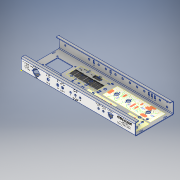
# Autodesk Inventor part: mainChassis
Saved by Autodesk Inventor 2018.3 (Build 223284000, 284)
## iProperties
Created: 2019-02-19
Part Number: mainChassis
Material: Aluminum 6061
Document SubType Name: Sheet Metal
Designer: RCCol
Density: 2.7 g/cm^3
Sheet Metal Rule: .125 thick aluminum
Appearance: Aluminum - Flat
Flat Pattern Width: 34.7497 cm
Flat Pattern Length: 60.325 cm
Flat Pattern Area: 2096.27 cm^2
Sheet Metal Width: 13.681 in
Sheet Metal Length: 23.750 in
Sheet Metal Area: 324.923 in^2
Author: RCCol
Autodesk Inventor part; units mm, degrees
ref_plane "YZ Plane" through (0, 0, 0) normal (1, 0, 0) x (0, 1, 0)
ref_plane "XZ Plane" through (0, 0, 0) normal (0, 1, 0) x (-1, 0, 0)
ref_plane "XY Plane" through (0, 0, 0) normal (0, 0, 1) x (1, 0, 0)
sketch "Sketch1" plane through (0, 0, 0) normal (0, 1, 0) x (-1, 0, 0)
  line L0 (0, 0) -> (-603.25, 0)
  line L1 (-603.25, 0) -> (-603.25, -204.47)
  line L2 (-603.25, -204.47) -> (0, -204.47)
  line L3 (0, -204.47) -> (0, 0)
  line L4 (0, 0) -> (-254, 0)
  line L5 (0, -79.375) -> (0, 0)
  dimension "d0" = 603.25
  dimension "d1" = 204.47
  constraints: 12 end point, 2 horizontal, 2 parallel, 1 perpendicular
  measures "d0" distance of L2.end L1.end
  measures "d1" distance of L1.end L0.end
extrude "Plate1" add sketch "Sketch1" along normal blind 3.175
sketch "Sketch2" plane through (0, 3.175, 0) normal (0, 1, 0) x (1, 0, 0)
  line L0 (41.3, 154.94) -> (117.45, 154.94)
  arc A0 (120.65, 151.74) -> (117.45, 154.94) centre (117.45, 151.74) ccw
  line L1 (41.3, 87.63) -> (117.45, 87.63)
  arc A1 (117.45, 87.63) -> (120.65, 90.83) centre (117.45, 90.83) ccw
  line L2 (38.1, 151.74) -> (38.1, 90.83)
  arc A2 (41.3, 154.94) -> (38.1, 151.74) centre (41.3, 151.74) ccw
  arc A3 (38.1, 90.83) -> (41.3, 87.63) centre (41.3, 90.83) ccw
  circle A4 centre (31.75, 177.5295) radius 1.5
  line L3 (120.65, 151.74) -> (120.65, 90.83)
  circle A5 centre (147.375, 75.2475) radius 1.65
  circle A6 centre (147.375, 164.1475) radius 1.65
  circle A7 centre (185.1575, 138.7475) radius 2.65
  circle A8 centre (185.1575, 178.435) radius 2.65
  circle A9 centre (235.9575, 87.1648) radius 2.65
  circle A10 centre (243.895, 87.1648) radius 2.65
  circle A11 centre (235.9575, 169.7148) radius 2.65
  circle A12 centre (243.895, 169.7148) radius 2.65
  circle A13 centre (259.135, 75.2475) radius 1.65
  circle A14 centre (259.135, 164.1475) radius 1.65
  circle A15 centre (551.549, 97.0569) radius 1.65
  arc A16 (187.6575, 169.4256) -> (182.6575, 169.4256) centre (185.1575, 169.4256) ccw
  arc A17 (182.6575, 164.4256) -> (187.6575, 164.4256) centre (185.1575, 164.4256) ccw
  line L4 (187.6575, 169.4256) -> (187.6575, 164.4256)
  line L5 (182.6575, 169.4256) -> (182.6575, 164.4256)
  arc A18 (187.6575, 90.4475) -> (182.6575, 90.4475) centre (185.1575, 90.4475) ccw
  arc A19 (182.6575, 85.4475) -> (187.6575, 85.4475) centre (185.1575, 85.4475) ccw
  line L6 (187.6575, 90.4475) -> (187.6575, 85.4475)
  line L7 (182.6575, 90.4475) -> (182.6575, 85.4475)
  arc A20 (308.1355, 175.935) -> (308.1355, 180.935) centre (308.1355, 178.435) ccw
  arc A21 (301.1355, 180.935) -> (301.1355, 175.935) centre (301.1355, 178.435) ccw
  line L8 (308.1355, 175.935) -> (301.1355, 175.935)
  line L9 (308.1355, 180.935) -> (301.1355, 180.935)
  arc A22 (243.048, 175.935) -> (243.048, 180.935) centre (243.048, 178.435) ccw
  arc A23 (236.048, 180.935) -> (236.048, 175.935) centre (236.048, 178.435) ccw
  line L10 (243.048, 175.935) -> (236.048, 175.935)
  line L11 (243.048, 180.935) -> (236.048, 180.935)
  arc A24 (298.195, 167.2148) -> (298.195, 172.2148) centre (298.195, 169.7148) ccw
  arc A25 (291.195, 172.2148) -> (291.195, 167.2148) centre (291.195, 169.7148) ccw
  line L12 (298.195, 167.2148) -> (291.195, 167.2148)
  line L13 (298.195, 172.2148) -> (291.195, 172.2148)
  arc A26 (308.1355, 110.435) -> (308.1355, 115.435) centre (308.1355, 112.935) ccw
  arc A27 (301.1355, 115.435) -> (301.1355, 110.435) centre (301.1355, 112.935) ccw
  line L14 (308.1355, 110.435) -> (301.1355, 110.435)
  line L15 (308.1355, 115.435) -> (301.1355, 115.435)
  arc A28 (308.1355, 99.735) -> (308.1355, 104.735) centre (308.1355, 102.235) ccw
  arc A29 (301.1355, 104.735) -> (301.1355, 99.735) centre (301.1355, 102.235) ccw
  line L16 (308.1355, 99.735) -> (301.1355, 99.735)
  line L17 (308.1355, 104.735) -> (301.1355, 104.735)
  arc A30 (243.048, 110.435) -> (243.048, 115.435) centre (243.048, 112.935) ccw
  arc A31 (236.048, 115.435) -> (236.048, 110.435) centre (236.048, 112.935) ccw
  line L18 (243.048, 110.435) -> (236.048, 110.435)
  line L19 (243.048, 115.435) -> (236.048, 115.435)
  arc A32 (243.048, 99.735) -> (243.048, 104.735) centre (243.048, 102.235) ccw
  arc A33 (236.048, 104.735) -> (236.048, 99.735) centre (236.048, 102.235) ccw
  line L20 (243.048, 99.735) -> (236.048, 99.735)
  line L21 (243.048, 104.735) -> (236.048, 104.735)
  arc A34 (298.195, 84.6648) -> (298.195, 89.6648) centre (298.195, 87.1648) ccw
  arc A35 (291.195, 89.6648) -> (291.195, 84.6648) centre (291.195, 87.1648) ccw
  line L22 (298.195, 84.6648) -> (291.195, 84.6648)
  line L23 (298.195, 89.6648) -> (291.195, 89.6648)
  circle A36 centre (237.6, 35.56) radius 15.1
  arc A37 (239.251, 57.4158) -> (238.6557, 58.0111) centre (238.6557, 57.4158) ccw
  arc A38 (238.6557, 53.1089) -> (239.251, 53.7042) centre (238.6557, 53.7042) ccw
  line L24 (239.251, 53.7042) -> (239.251, 57.4158)
  arc A39 (236.5443, 58.0111) -> (235.949, 57.4158) centre (236.5443, 57.4158) ccw
  line L25 (235.949, 53.7042) -> (235.949, 57.4158)
  line L26 (238.6557, 58.0111) -> (236.5443, 58.0111)
  line L27 (238.6557, 53.1089) -> (236.5443, 53.1089)
  arc A40 (235.949, 53.7042) -> (236.5443, 53.1089) centre (236.5443, 53.7042) ccw
  arc A41 (239.251, 17.4158) -> (238.6557, 18.0111) centre (238.6557, 17.4158) ccw
  arc A42 (238.6557, 13.1089) -> (239.251, 13.7042) centre (238.6557, 13.7042) ccw
  line L28 (239.251, 13.7042) -> (239.251, 17.4158)
  arc A43 (236.5443, 18.0111) -> (235.949, 17.4158) centre (236.5443, 17.4158) ccw
  line L29 (235.949, 13.7042) -> (235.949, 17.4158)
  line L30 (238.6557, 18.0111) -> (236.5443, 18.0111)
  line L31 (238.6557, 13.1089) -> (236.5443, 13.1089)
  arc A44 (235.949, 13.7042) -> (236.5443, 13.1089) centre (236.5443, 13.7042) ccw
  circle A45 centre (174.1, 35.56) radius 15.1
  arc A46 (175.751, 57.4158) -> (175.1557, 58.0111) centre (175.1557, 57.4158) ccw
  arc A47 (175.1557, 53.1089) -> (175.751, 53.7042) centre (175.1557, 53.7042) ccw
  line L32 (175.751, 53.7042) -> (175.751, 57.4158)
  arc A48 (173.0443, 58.0111) -> (172.449, 57.4158) centre (173.0443, 57.4158) ccw
  line L33 (172.449, 53.7042) -> (172.449, 57.4158)
  line L34 (175.1557, 58.0111) -> (173.0443, 58.0111)
  line L35 (175.1557, 53.1089) -> (173.0443, 53.1089)
  arc A49 (172.449, 53.7042) -> (173.0443, 53.1089) centre (173.0443, 53.7042) ccw
  arc A50 (175.751, 17.4158) -> (175.1557, 18.0111) centre (175.1557, 17.4158) ccw
  arc A51 (175.1557, 13.1089) -> (175.751, 13.7042) centre (175.1557, 13.7042) ccw
  line L36 (175.751, 13.7042) -> (175.751, 17.4158)
  arc A52 (173.0443, 18.0111) -> (172.449, 17.4158) centre (173.0443, 17.4158) ccw
  line L37 (172.449, 13.7042) -> (172.449, 17.4158)
  line L38 (175.1557, 18.0111) -> (173.0443, 18.0111)
  line L39 (175.1557, 13.1089) -> (173.0443, 13.1089)
  arc A53 (172.449, 13.7042) -> (173.0443, 13.1089) centre (173.0443, 13.7042) ccw
  circle A54 centre (110.6, 35.56) radius 15.1
  arc A55 (112.251, 57.4158) -> (111.6557, 58.0111) centre (111.6557, 57.4158) ccw
  arc A56 (111.6557, 53.1089) -> (112.251, 53.7042) centre (111.6557, 53.7042) ccw
  line L40 (112.251, 53.7042) -> (112.251, 57.4158)
  arc A57 (109.5443, 58.0111) -> (108.949, 57.4158) centre (109.5443, 57.4158) ccw
  line L41 (108.949, 53.7042) -> (108.949, 57.4158)
  line L42 (111.6557, 58.0111) -> (109.5443, 58.0111)
  line L43 (111.6557, 53.1089) -> (109.5443, 53.1089)
  arc A58 (108.949, 53.7042) -> (109.5443, 53.1089) centre (109.5443, 53.7042) ccw
  arc A59 (112.251, 17.4158) -> (111.6557, 18.0111) centre (111.6557, 17.4158) ccw
  arc A60 (111.6557, 13.1089) -> (112.251, 13.7042) centre (111.6557, 13.7042) ccw
  line L44 (112.251, 13.7042) -> (112.251, 17.4158)
  arc A61 (109.5443, 18.0111) -> (108.949, 17.4158) centre (109.5443, 17.4158) ccw
  line L45 (108.949, 13.7042) -> (108.949, 17.4158)
  line L46 (111.6557, 18.0111) -> (109.5443, 18.0111)
  line L47 (111.6557, 13.1089) -> (109.5443, 13.1089)
  arc A62 (108.949, 13.7042) -> (109.5443, 13.1089) centre (109.5443, 13.7042) ccw
  circle A63 centre (47.1, 35.56) radius 15.1
  arc A64 (48.751, 57.4158) -> (48.1557, 58.0111) centre (48.1557, 57.4158) ccw
  arc A65 (48.1557, 53.1089) -> (48.751, 53.7042) centre (48.1557, 53.7042) ccw
  line L48 (48.751, 53.7042) -> (48.751, 57.4158)
  arc A66 (46.0443, 58.0111) -> (45.449, 57.4158) centre (46.0443, 57.4158) ccw
  line L49 (45.449, 53.7042) -> (45.449, 57.4158)
  line L50 (48.1557, 58.0111) -> (46.0443, 58.0111)
  line L51 (48.1557, 53.1089) -> (46.0443, 53.1089)
  arc A67 (45.449, 53.7042) -> (46.0443, 53.1089) centre (46.0443, 53.7042) ccw
  arc A68 (48.751, 17.4158) -> (48.1557, 18.0111) centre (48.1557, 17.4158) ccw
  arc A69 (48.1557, 13.1089) -> (48.751, 13.7042) centre (48.1557, 13.7042) ccw
  line L52 (48.751, 13.7042) -> (48.751, 17.4158)
  arc A70 (46.0443, 18.0111) -> (45.449, 17.4158) centre (46.0443, 17.4158) ccw
  line L53 (45.449, 13.7042) -> (45.449, 17.4158)
  line L54 (48.1557, 18.0111) -> (46.0443, 18.0111)
  line L55 (48.1557, 13.1089) -> (46.0443, 13.1089)
  arc A71 (45.449, 13.7042) -> (46.0443, 13.1089) centre (46.0443, 13.7042) ccw
  circle A72 centre (159.7575, 106.3403) radius 4.8
  circle A73 centre (212.2, 93.5148) radius 4.8
  circle A74 centre (309.5568, 135.335) radius 6.35
  circle A75 centre (234.6268, 135.335) radius 6.35
  circle A76 centre (269.35, 26.9408) radius 1.651
  circle A77 centre (515.9375, 36.5125) radius 9.525
  circle A78 centre (515.3168, 50.7865) radius 1.651
  circle A79 centre (516.5582, 22.2385) radius 1.651
  circle A80 centre (530.225, 142.875) radius 9.525
  circle A81 centre (530.225, 157.1625) radius 1.651
  circle A82 centre (530.225, 128.5875) radius 1.651
  circle A83 centre (425.45, 142.875) radius 9.525
  circle A84 centre (425.45, 157.1625) radius 1.651
  circle A85 centre (425.45, 128.5875) radius 1.651
  circle A86 centre (363.5375, 142.875) radius 9.525
  circle A87 centre (363.5375, 157.1625) radius 1.651
  circle A88 centre (363.5375, 128.5875) radius 1.651
  circle A89 centre (336.55, 37.1475) radius 9.525
  circle A90 centre (336.757, 22.8615) radius 1.651
  circle A91 centre (336.343, 51.4335) radius 1.651
  circle A92 centre (205.85, 26.9408) radius 1.651
  circle A93 centre (78.85, 26.9408) radius 1.651
  circle A94 centre (78.85, 63.0879) radius 1.651
  circle A95 centre (19.05, 63.0879) radius 1.651
  circle A96 centre (142.35, 26.035) radius 1.651
  circle A97 centre (22.225, 20.5908) radius 1.651
  arc A98 (187.6575, 104.4569) -> (182.6575, 104.4569) centre (185.1575, 104.4569) ccw
  arc A99 (182.6575, 99.4569) -> (187.6575, 99.4569) centre (185.1575, 99.4569) ccw
  line L56 (187.6575, 104.4569) -> (187.6575, 99.4569)
  line L57 (182.6575, 104.4569) -> (182.6575, 99.4569)
  circle A100 centre (193.85, 60.5908) radius 1.65
  circle A101 centre (217.85, 60.5908) radius 1.65
  circle A102 centre (205.85, 60.5908) radius 4.826
  circle A103 centre (137.16, 62.3578) radius 1.651
  circle A104 centre (558.8, 109.5375) radius 4.826
  circle A105 centre (558.8, 84.1375) radius 4.826
  circle A106 centre (518.6157, 61.2782) radius 2.3813
  circle A107 centre (529.5939, 97.3765) radius 6.35
  circle A108 centre (563.0654, 61.4489) radius 2.3813
  circle A109 centre (31.75, 159.385) radius 3.175
  circle A110 centre (127, 159.385) radius 3.175
  circle A111 centre (31.75, 83.185) radius 3.175
  circle A112 centre (127, 83.185) radius 3.175
  circle A113 centre (565.8874, 37.1475) radius 9.525
  circle A114 centre (565.8026, 51.4347) radius 1.651
  circle A115 centre (565.9721, 22.8603) radius 1.651
  circle A116 centre (78.85, 35.56) radius 3.2385
  circle A117 centre (142.35, 35.56) radius 3.2385
  circle A118 centre (205.85, 35.56) radius 3.2385
  circle A119 centre (269.35, 35.56) radius 3.2385
  circle A120 centre (6.35, 165.735) radius 2.667
  circle A121 centre (6.35, 158.3944) radius 1.5875
  circle A122 centre (6.35, 173.0756) radius 1.5875
  circle A123 centre (6.35, 38.735) radius 2.667
  circle A124 centre (6.35, 31.3944) radius 1.5875
  circle A125 centre (6.35, 46.0756) radius 1.5875
  circle A126 centre (596.9, 38.735) radius 2.667
  circle A127 centre (596.9, 46.0756) radius 1.5875
  circle A128 centre (596.9, 31.3944) radius 1.5875
  circle A129 centre (596.9, 165.735) radius 2.667
  circle A130 centre (596.9, 173.0756) radius 1.5875
  circle A131 centre (596.9, 158.3944) radius 1.5875
  circle A132 centre (257.175, 61.9125) radius 3.2385
  circle A133 centre (117.45, 90.83) radius 3.2
  circle A134 centre (41.3, 90.83) radius 3.2
  circle A135 centre (41.3, 151.74) radius 3.2
  circle A136 centre (117.45, 151.74) radius 3.2
  line L58 (117.45, 87.63) -> (41.3, 87.63)
  line L59 (41.3, 87.63) -> (41.3, 154.94)
  line L60 (41.3, 154.94) -> (117.45, 154.94)
  line L61 (117.45, 154.94) -> (117.45, 87.63)
  line L62 (38.1, 90.83) -> (120.65, 90.83)
  line L63 (120.65, 90.83) -> (120.65, 151.74)
  line L64 (120.65, 151.74) -> (38.1, 151.74)
  line L65 (38.1, 151.74) -> (38.1, 90.83)
  line L66 (481.5672, 92.8982) -> (586.4692, 92.8982) construction
  line L67 (586.4692, 92.8982) -> (586.4692, 13.4373) construction
  line L68 (586.4692, 13.4373) -> (481.5672, 13.4373) construction
  line L69 (481.5672, 13.4373) -> (481.5672, 92.8982) construction
  line L70 (327.7837, 182.0084) -> (581.4999, 182.0084) construction
  line L71 (581.4999, 182.0084) -> (581.4999, 102.7644) construction
  line L72 (581.4999, 102.7644) -> (327.7837, 102.7644) construction
  line L73 (327.7837, 102.7644) -> (327.7837, 182.0084) construction
  line L74 (264.3245, 93.0716) -> (416.75, 93.5014) construction
  line L75 (416.75, 93.5014) -> (416.9742, 13.9788) construction
  line L76 (416.9742, 13.9788) -> (264.5487, 13.549) construction
  line L77 (264.5487, 13.549) -> (264.3245, 93.0716) construction
  circle A137 centre (298.195, 37.1475) radius 9.525
  circle A138 centre (298.3621, 51.434) radius 1.651
  circle A139 centre (298.0279, 22.861) radius 1.651
  line L78 (137.2091, 179.1073) -> (295.4903, 179.1073) construction
  line L79 (295.4903, 179.1073) -> (295.4903, 100.0089) construction
  line L80 (295.4903, 100.0089) -> (137.2091, 100.0089) construction
  line L81 (137.2091, 100.0089) -> (137.2091, 179.1073) construction
  circle A140 centre (436.5625, 46.0375) radius 14.9987
  circle A141 centre (436.5625, 68.8975) radius 1.651
  circle A142 centre (436.5625, 23.1775) radius 1.651
  dimension "JacobiRadiusSize" = 3.175
  dimension "d353" = 29.9974
  dimension "d378" = 3.302
  dimension "d379" = 3.302
  dimension "d417" = 22.86
  dimension "d418" = 22.86
  constraints: 141 centre point, 132 end point, 116 point on circle, 4 coincident, 4 parallel, 2 horizontal, 2 horizontal alignment, 2 perpendicular, 2 point on line, 12 other
  measures "d353" diameter of A140
  measures "d378" diameter of A141
  measures "d379" diameter of A142
  measures "d417" distance of A141.centre A140.centre
  measures "d418" distance of A140.centre A142.centre
extrude "Cut1" cut sketch "Sketch2" against normal blind 3.175 contours L59 L64 A2 | L0 A136 L64 A135 | A135 L64 L59 | L61 L64 A136 | A0 L64 L61 | A135 L59 A134 L2 | L64 L59 A135 | L64 A136 L61 A133 L62 A134 L59 A135 | A135 L59 L64 | L3 A133 L61 A136 | A136 L61 L64 | L64 L61 A136 | L62 L59 A3 | A134 L59 L62 | L62 L61 A133 | A1 L61 L62 | A134 L62 A133 L1 | L59 L62 A134 | A134 L62 L59 | A133 L62 L61 | L61 L62 A133 | A5 | A6 | A7 | A8 | A9 | A10 | A11 | A12 | A13 | A14 | A15 | L4 A17 L5 A16 | L6 A19 L7 A18 | L8 A21 L9 A20 | L10 A23 L11 A22 | L12 A25 L13 A24 | L14 A27 L15 A26 | L16 A29 L17 A28 | L18 A31 L19 A30 | L20 A33 L21 A32 | L22 A35 L23 A34 | A36 | L24 A38 L27 A40 L25 A39 L26 A37 | L28 A42 L31 A44 L29 A43 L30 A41 | A45 | L32 A47 L35 A49 L33 A48 L34 A46 | L36 A51 L39 A53 L37 A52 L38 A50 | A54 | L40 A56 L43 A58 L41 A57 L42 A55 | L44 A60 L47 A62 L45 A61 L46 A59 | A63 | L48 A65 L51 A67 L49 A66 L50 A64 | L52 A69 L55 A71 L53 A70 L54 A68 | A72 | A73 | A74 | A75 | A76 | A77 | A78 | A79 | A80 | A81 | A82 | A83 | A84 | A85 | A86 | A87 | A88 | A89 | A90 | A91 | A92 | A93 | A94 | A95 | A96 | A97 | L56 A99 L57 A98 | A100 | A101 | A102 | A103 | A104 | A105 | A106 | A107 | A108 | A109 | A110 | A111 | A112 | A113 | A114 | A115 | A116 | A117 | A118 | A119 | A120 | A121 | A122 | A123 | A124 | A125 | A126 | A127 | A128 | A129 | A130 | A131 | A132 | A137 | A138 | A139 | A140 | A141 | A142
sketch "Sketch3" plane through (603.25, 0, -3.175) normal (0, 0, 1) x (1, 0, 0)
  line L0 (-603.25, 0) -> (0, 0)
  line L1 (0, 0) -> (0, 63.5)
  line L2 (0, 63.5) -> (-603.25, 63.5)
  line L3 (-603.25, 63.5) -> (-603.25, 0)
  constraints: 6 end point, 1 horizontal, 1 perpendicular, 1 vertical
edge flange "Flange1" height 63.5 angle 90 thickness 3.175 bend radius 3.175 thickness toward (0, 0, 1) relief straight relief width 3.175 relief depth 1.5875 edges at (301.625, 3.175, 0) wall of the first edge with corners at (0, 0, -3.175) (603.25, 0, -3.175) (603.25, 63.5, -3.175) (0, 63.5, -3.175)
bend "Bend1"
corner "Corner1"
sketch "Sketch4" plane through (603.25, 60.325, 0) normal (0, 1, 0) x (-1, 0, 0)
  line L0 (603.25, 0) -> (0, 0)
  line L1 (0, 0) -> (0, -19.05)
  line L2 (0, -19.05) -> (603.25, -19.05)
  line L3 (603.25, -19.05) -> (603.25, 0)
  constraints: 6 end point, 1 horizontal, 1 perpendicular, 1 vertical
edge flange "Flange2" height 19.05 angle 90 thickness 3.175 bend radius 3.175 thickness toward (0, 1, 0) relief straight relief width 3.175 relief depth 1.5875 edges at (301.625, 63.5, -3.175) wall of the first edge with corners at (0, 60.325, 0) (603.25, 60.325, 0) (603.25, 60.325, -19.05) (0, 60.325, -19.05)
bend "Bend2"
corner "Corner2"
sketch "Sketch5" plane through (0, 6.35, 0) normal (0, 0, 1) x (1, 0, 0)
  circle A0 centre (78.85, 25.4) radius 17.4625
  circle A1 centre (99.805, 25.4) radius 1.778
  circle A2 centre (57.895, 25.4) radius 1.778
  line L0 (148.065, 22.0907) -> (148.065, 28.7093)
  line L1 (136.635, 22.0907) -> (136.635, 28.7093)
  arc A3 (136.635, 22.0907) -> (148.065, 22.0907) centre (142.35, 25.4) ccw
  arc A4 (148.065, 28.7093) -> (136.635, 28.7093) centre (142.35, 25.4) ccw
  line L2 (193.9018, 20.2386) -> (192.3982, 20.2386)
  arc A5 (193.9018, 19.2226) -> (192.3982, 19.2226) centre (193.15, 25.4) ccw
  line L3 (192.3982, 20.2386) -> (192.3982, 19.2226)
  line L4 (193.9018, 19.2226) -> (193.9018, 20.2386)
  line L5 (219.3018, 20.2386) -> (217.7982, 20.2386)
  arc A6 (219.3018, 19.2226) -> (217.7982, 19.2226) centre (218.55, 25.4) ccw
  line L6 (217.7982, 20.2386) -> (217.7982, 19.2226)
  line L7 (219.3018, 19.2226) -> (219.3018, 20.2386)
  circle A7 centre (261.3213, 25.4) radius 4.7625
  circle A8 centre (286.7213, 25.4) radius 4.7625
  circle A9 centre (312.1213, 25.4) radius 4.7625
  circle A10 centre (409.575, 25.5399) radius 4.7625
  circle A11 centre (434.975, 25.5399) radius 4.7625
  circle A12 centre (473.075, 25.5399) radius 12.1031
  circle A13 centre (460.2734, 32.9821) radius 1.778
  circle A14 centre (485.8766, 32.9821) radius 1.778
  circle A15 centre (473.075, 10.7317) radius 1.778
  line L8 (136.635, 28.7093) -> (148.065, 28.7093)
  line L9 (148.065, 28.7093) -> (148.065, 22.0907)
  line L10 (148.065, 22.0907) -> (136.635, 22.0907)
  line L11 (136.635, 22.0907) -> (136.635, 28.7093)
  arc A16 (148.065, 28.7093) -> (136.635, 28.7093) centre (142.35, 25.4) ccw
  arc A17 (136.635, 22.0907) -> (148.065, 22.0907) centre (142.35, 25.4) ccw
  arc A18 (136.635, 22.0907) -> (148.065, 22.0907) centre (142.35, 25.4) ccw
  arc A19 (193.9018, 19.2226) -> (192.3982, 19.2226) centre (193.15, 25.4) ccw
  line L12 (193.9018, 19.2226) -> (193.9018, 20.2386)
  line L13 (192.3982, 20.2386) -> (192.3982, 19.2226)
  point P0 (0, -6.35)
  dimension "JacobiRadiusSize" = 3.175
  constraints: 28 end point, 23 point on circle, 20 centre point, 5 point on line, 2 parallel, 1 concentric, 1 horizontal, 1 perpendicular, 1 vertical
extrude "Cut2" cut sketch "Sketch5" against normal blind 3.175
sketch "Sketch6" plane through (0, 0, -201.295) normal (0, 0, -1) x (-1, 0, 0)
  line L0 (-603.25, 0) -> (0, 0)
  line L1 (0, 0) -> (0, 63.5)
  line L2 (0, 63.5) -> (-603.25, 63.5)
  line L3 (-603.25, 63.5) -> (-603.25, 0)
  constraints: 6 end point, 1 horizontal, 1 perpendicular, 1 vertical
edge flange "Flange3" height 63.5 angle 90 thickness 3.175 bend radius 3.175 thickness toward (0, 0, -1) relief straight relief width 3.175 relief depth 1.5875 edges at (301.625, 3.175, -204.47) wall of the first edge with corners at (603.25, 0, -201.295) (0, 0, -201.295) (0, 63.5, -201.295) (603.25, 63.5, -201.295)
bend "Bend3"
corner "Corner3"
sketch "Sketch7" plane through (0, 60.325, -204.47) normal (0, 1, 0) x (-1, 0, 0)
  line L0 (-603.25, 0) -> (0, 0)
  line L1 (0, 0) -> (0, 19.05)
  line L2 (0, 19.05) -> (-603.25, 19.05)
  line L3 (-603.25, 19.05) -> (-603.25, 0)
  constraints: 6 end point, 1 horizontal, 1 perpendicular, 1 vertical
edge flange "Flange4" height 19.05 angle 90 thickness 3.175 bend radius 3.175 thickness toward (0, 1, 0) relief straight relief width 3.175 relief depth 1.5875 edges at (301.625, 63.5, -201.295) wall of the first edge with corners at (603.25, 60.325, -204.47) (0, 60.325, -204.47) (0, 60.325, -185.42) (603.25, 60.325, -185.42)
bend "Bend4"
corner "Corner4"
sketch "Sketch8" plane through (603.25, 6.35, -204.47) normal (0, 0, -1) x (-1, 0, 0)
  line L0 (0, -6.35) -> (603.25, -6.35)
  line L1 (603.25, -6.35) -> (603.25, 57.15)
  line L2 (603.25, 57.15) -> (0, 57.15)
  line L3 (0, 57.15) -> (0, -6.35)
  circle A0 centre (31.9541, 38.1) radius 4.7625
  circle A1 centre (70.0541, 25.4) radius 4.7625
  circle A2 centre (190.9581, 25.4) radius 4.7625
  circle A3 centre (305.2581, 25.4) radius 4.7625
  circle A4 centre (444.9581, 25.4) radius 4.7625
  circle A5 centre (394.1581, 25.4) radius 4.7625
  circle A6 centre (356.0581, 25.4) radius 4.7625
  circle A7 centre (267.1581, 25.4) radius 4.7625
  circle A8 centre (229.0581, 25.4) radius 4.7625
  circle A9 centre (152.8581, 25.4) radius 4.7625
  circle A10 centre (31.9541, 12.7) radius 4.7625
  circle A11 centre (31.9541, 12.7) radius 4.7625
  circle A12 centre (152.8581, 25.4) radius 4.7625
  circle A13 centre (229.0581, 25.4) radius 4.7625
  circle A14 centre (267.1581, 25.4) radius 4.7625
  circle A15 centre (356.0581, 25.4) radius 4.7625
  circle A16 centre (394.1581, 25.4) radius 4.7625
  circle A17 centre (444.9581, 25.4) radius 4.7625
  circle A18 centre (305.2581, 25.4) radius 4.7625
  circle A19 centre (190.9581, 25.4) radius 4.7625
  circle A20 centre (70.0541, 25.4) radius 4.7625
  circle A21 centre (31.9541, 38.1) radius 4.7625
  circle A22 centre (571.5, 25.4) radius 3.9624
  circle A23 centre (95.4541, 39.6875) radius 1.7272
  circle A24 centre (95.4541, 11.1125) radius 1.7272
  line L4 (91.4854, 18.2562) -> (91.4854, 32.5437)
  line L5 (91.4854, 32.5437) -> (99.4229, 32.5438)
  line L6 (99.4229, 32.5438) -> (99.4229, 18.2563)
  line L7 (99.4229, 18.2563) -> (91.4854, 18.2562)
  circle A25 centre (111.4561, 39.6875) radius 1.7272
  circle A26 centre (111.4561, 11.1125) radius 1.7272
  line L8 (107.4874, 18.2562) -> (107.4874, 32.5437)
  line L9 (107.4874, 32.5437) -> (115.4249, 32.5438)
  line L10 (115.4249, 32.5438) -> (115.4249, 18.2563)
  line L11 (115.4249, 18.2563) -> (107.4874, 18.2562)
  circle A27 centre (127.4581, 39.6875) radius 1.7272
  circle A28 centre (127.4581, 11.1125) radius 1.7272
  line L12 (123.4894, 18.2562) -> (123.4894, 32.5437)
  line L13 (123.4894, 32.5437) -> (131.4269, 32.5438)
  line L14 (131.4269, 32.5438) -> (131.4269, 18.2563)
  line L15 (131.4269, 18.2563) -> (123.4894, 18.2562)
  circle A29 centre (330.6581, 39.6875) radius 1.7272
  circle A30 centre (330.6581, 11.1125) radius 1.7272
  line L16 (326.6894, 18.2562) -> (326.6894, 32.5437)
  line L17 (326.6894, 32.5437) -> (334.6269, 32.5438)
  line L18 (334.6269, 32.5438) -> (334.6269, 18.2563)
  line L19 (334.6269, 18.2563) -> (326.6894, 18.2562)
  circle A31 centre (419.5581, 39.6875) radius 1.7272
  circle A32 centre (419.5581, 11.1125) radius 1.7272
  line L20 (415.5894, 18.2562) -> (415.5894, 32.5437)
  line L21 (415.5894, 32.5437) -> (423.5269, 32.5438)
  line L22 (423.5269, 32.5438) -> (423.5269, 18.2563)
  line L23 (423.5269, 18.2563) -> (415.5894, 18.2562)
  dimension "JacobiRadiusSize" = 3.175
  constraints: 48 end point, 33 centre point
extrude "Cut3" cut sketch "Sketch8" against normal blind 3.175 contours A0 | A1 | A2 | A3 | A4 | A5 | A6 | A7 | A8 | A9 | A10 | A22 | A23 | A24 | L4 L5 L6 L7 | A25 | A26 | L8 L9 L10 L11 | A27 | A28 | L12 L13 L14 L15 | A29 | A30 | L16 L17 L18 L19 | A31 | A32 | L20 L21 L22 L23
sketch "Sketch9" plane through (603.25, 6.35, -204.47) normal (0, 0, -1) x (-1, 0, 0)
  line L0 (0, 50.8) -> (0, 53.975) projected
  line L1 (0, 53.975) -> (603.25, 53.975) projected
  line L2 (603.25, 53.975) -> (0, 53.975) projected
  line L3 (0, 50.8) -> (0, 0) projected
  line L4 (0, 50.8) -> (0, 0) projected
  line L5 (0, 50.8) -> (603.2512, 50.8) construction
  line L6 (603.2512, 50.8) -> (603.2512, -0.0001) construction
  line L7 (603.2512, -0.0001) -> (0, -0.0001) construction
  line L8 (0, -0.0001) -> (0, 50.8) construction
  point P0 (603.25, -6.35)
  constraints: 2 other
decal "Decal1"
sketch "Sketch10" plane through (0, 6.35, 0) normal (0, 0, 1) x (1, 0, 0)
  line L0 (0, 53.975) -> (0, 50.8) projected
  line L1 (0, 53.975) -> (603.2512, 53.975) construction
  line L2 (603.2512, 53.975) -> (603.2512, -3.1751) construction
  line L3 (603.2512, -3.1751) -> (0, -3.1751) construction
  line L4 (0, -3.1751) -> (0, 53.975) construction
  point P0 (0, -6.35)
  constraints: 2 other
decal "Decal2"
sketch "Sketch11" plane through (0, 3.175, 0) normal (0, 1, 0) x (1, 0, 0)
  line L0 (327.7837, 182.0084) -> (581.4999, 182.0084) construction
  line L1 (581.4999, 182.0084) -> (581.4999, 102.7644) construction
  line L2 (581.4999, 102.7644) -> (327.7837, 102.7644) construction
  line L3 (327.7837, 102.7644) -> (327.7837, 182.0084) construction
  line L4 (137.2091, 179.1073) -> (295.4903, 179.1073) construction
  line L5 (295.4903, 179.1073) -> (295.4903, 100.0089) construction
  line L6 (295.4903, 100.0089) -> (137.2091, 100.0089) construction
  line L7 (137.2091, 100.0089) -> (137.2091, 179.1073) construction
  line L8 (481.5672, 92.8982) -> (586.4692, 92.8982) construction
  line L9 (586.4692, 92.8982) -> (586.4692, 13.4373) construction
  line L10 (586.4692, 13.4373) -> (481.5672, 13.4373) construction
  line L11 (481.5672, 13.4373) -> (481.5672, 92.8982) construction
  point P0 (0, 0)
  constraints: 6 other
decal "Decal3"
decal "Decal4"
decal "Decal5"
decal "Decal6"
equation "\"JacobiRadiusSize\" = BendRadius"
equation "\"d3\" = Thickness"
equation "\"d27\" = Thickness"
equation "\"d49\" = Thickness"
equation "\"d2\" = Thickness"
equation "\"d5\" = BendReliefWidth"
equation "\"d6\" = BendReliefDepth"
equation "\"d7\" = MinimumRemnant"
equation "\"d8\" = TransitionRadius"
equation "\"d11\" = BendRadius"
equation "\"d12\" = CornerReliefSize"
equation "\"d13\" = GapSize"
equation "\"d14\" = JacobiRadiusSize"
equation "\"d17\" = BendReliefWidth"
equation "\"d18\" = BendReliefDepth"
equation "\"d19\" = MinimumRemnant"
equation "\"d20\" = TransitionRadius"
equation "\"d23\" = BendRadius"
equation "\"d24\" = CornerReliefSize"
equation "\"d25\" = GapSize"
equation "\"d26\" = JacobiRadiusSize"
equation "\"d29\" = BendReliefWidth"
equation "\"d30\" = BendReliefDepth"
equation "\"d31\" = MinimumRemnant"
equation "\"d32\" = TransitionRadius"
equation "\"d35\" = BendRadius"
equation "\"d36\" = CornerReliefSize"
equation "\"d37\" = GapSize"
equation "\"d38\" = JacobiRadiusSize"
equation "\"d39\" = BendReliefWidth"
equation "\"d40\" = BendReliefDepth"
equation "\"d41\" = MinimumRemnant"
equation "\"d42\" = TransitionRadius"
equation "\"d45\" = BendRadius"
equation "\"d46\" = CornerReliefSize"
equation "\"d47\" = GapSize"
equation "\"d48\" = JacobiRadiusSize"
equation "\"BendRadius\" = Thickness"
equation "\"BendReliefWidth\" = Thickness"
equation "\"BendReliefDepth\" = 0.5 * Thickness"
equation "\"CornerReliefSize\" = 4 * Thickness"
equation "\"MinimumRemnant\" = 2 * Thickness"
equation "\"TransitionRadius\" = BendRadius"
equation "\"GapSize\" = Thickness"
equation "\"Thickness\" = 3.175"
body "Solid1"
